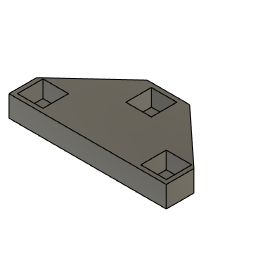
tripodmount v1 (Autodesk Fusion 360 design; units mm, degrees)
Autodesk Fusion 360 part; units mm, degrees
sketch "Sketch1" plane through (0, 0, 0) normal (0, 0, 1) x (1, 0, 0)
  line L0 (0, 0) -> (74, 0)
  line L1 (0, 0) -> (0, 13)
  line L2 (37, 0) -> (37, 38) construction
  line L3 (37, 38) -> (27, 38)
  line L4 (0, 13) -> (27, 38)
  line L5 (37, 38) -> (47, 38)
  line L6 (74, 0) -> (74, 13)
  line L7 (74, 13) -> (47, 38)
  dimension "d1" = 74
  dimension "d2" = 13
  dimension "d3" = 38
  dimension "d4" = 10
  dimension "d5" = 10
  dimension "d6" = 13
  constraint coincident L0.start L1.start
  constraint horizontal L0
  constraint perpendicular L0 L1
  constraint midpoint L0 L2.start
  constraint perpendicular L0 L2
  constraint perpendicular L2 L3
  constraint perpendicular L2 L5
  constraint perpendicular L0 L6
  measures "d1" distance of L0.start L0.end
  measures "d2" distance of L0.start L1.end
  measures "d3" distance of L2.start L2.end
  measures "d4" distance of L2.end L3.end
  measures "d5" distance of L2.end L5.end
  measures "d6" distance of L0.end L6.end
extrude "Extrude1" add sketch "Sketch1" along normal blind 10
sketch "Sketch2" plane through (0, 0, 10) normal (0, 0, 1) x (-1, 0, 0)
  line L0 (0, 0) -> (-74, 0)
  line L1 (-74, 0) -> (-74, -13)
  line L2 (-74, -13) -> (-47, -38)
  line L3 (-47, -38) -> (-27, -38)
  line L4 (-27, -38) -> (0, -13)
  line L5 (0, -13) -> (0, 0)
  line L6 (-37, -36) -> (-31, -36) construction
  line L7 (0, 0) -> (-2, 0) construction
  line L8 (-2, 0) -> (-2, -2) construction
  line L9 (-74, 0) -> (-72, 0) construction
  line L10 (-72, 0) -> (-72, -2) construction
  line L11 (-31, -36) -> (-43, -36)
  line L12 (-43, -36) -> (-43, -24)
  line L13 (-43, -24) -> (-31, -24)
  line L14 (-31, -24) -> (-31, -36)
  line L15 (-2, -2) -> (-14, -2)
  line L16 (-14, -2) -> (-14, -14)
  line L17 (-14, -14) -> (-2, -14)
  line L18 (-2, -14) -> (-2, -2)
  line L19 (-72, -2) -> (-60, -2)
  line L20 (-60, -2) -> (-60, -14)
  line L21 (-60, -14) -> (-72, -14)
  line L22 (-72, -14) -> (-72, -2)
  dimension "d10" = 6
  dimension "d11" = 2
  dimension "d12" = 2
  dimension "d13" = 2
  dimension "d14" = 2
  dimension "d15" = 12
  dimension "d16" = 12
  dimension "d17" = 12
  dimension "d18" = 12
  dimension "d19" = 12
  dimension "d20" = 12
  constraint coincident L0.start L5.end
  constraint perpendicular L5 L7
  constraint perpendicular L7 L8
  constraint coincident L0.end L1.start
  constraint perpendicular L1 L9
  constraint perpendicular L0 L10
  constraint horizontal L11
  constraint vertical L12
  constraint horizontal L13
  constraint vertical L14
  constraint horizontal L15
  constraint vertical L16
  constraint horizontal L17
  constraint vertical L18
  constraint horizontal L19
  constraint vertical L20
  constraint horizontal L21
  constraint vertical L22
  measures "d10" distance of L6.start L6.end
  measures "d11" distance of L0.start L7.end
  measures "d12" distance of L7.end L8.end
  measures "d13" distance of L0.end L9.end
  measures "d14" distance of L9.end L10.end
  measures "d15" distance of L6.end L11.end
  measures "d16" distance of L6.end L13.end
  measures "d17" distance of L8.end L15.end
  measures "d18" distance of L8.end L17.end
  measures "d19" distance of L10.end L19.end
  measures "d20" distance of L10.end L21.end
extrude "Extrude2" cut sketch "Sketch2" against normal blind 8 contours L11 L12 L13 L14 | L15 L16 L17 L18 | L19 L20 L21 L22
